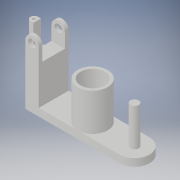
# Autodesk Inventor part: ValveBaseMk2.5
Saved by Autodesk Inventor 2019 (Build 230136000, 136)
## iProperties
Created: 2019-01-19
Part Number: ValveBaseMk2.5
Material: Generic
Document SubType Name: Modeling
Designer: Kepler
Density: 1 g/cm^3
Appearance: Default
Author: Kepler
Autodesk Inventor part; units mm, degrees
ref_plane "YZ Plane" through (0, 0, 0) normal (1, 0, 0) x (0, 1, 0)
ref_plane "XZ Plane" through (0, 0, 0) normal (0, 1, 0) x (-1, 0, 0)
ref_plane "XY Plane" through (0, 0, 0) normal (0, 0, 1) x (1, 0, 0)
sketch "Sketch1" plane through (0, 0, 0) normal (0, 0, 1) x (1, 0, 0)
  line L0 (0, 0) -> (0, 40)
  line L1 (0, 0) -> (63, 0)
  line L2 (63, 0) -> (63, 5)
  line L3 (63, 5) -> (9, 5)
  arc A0 (9, 40) -> (0, 40) centre (4.5, 40) ccw
  line L4 (9, 40) -> (9, 5)
  circle A1 centre (4.5, 40) radius 2.5
  dimension "d0" = 40
  dimension "d2" = 5
  dimension "d6" = 4.5
  dimension "d7" = 5
  dimension "d8" = 9
  dimension "d9" = 54
  dimension "d47" = 32.5
  constraints: 10 end point, 3 perpendicular, 2 centre point, 2 point on circle, 2 tangent, 1 coincident, 1 horizontal, 1 vertical
  measures "d0" distance of L0.start L0.end
  measures "d2" distance of L1.end L2.end
  measures "d6" radius of A0
  measures "d7" diameter of A1
  measures "d8" distance between parallel lines of L4 L0
  measures "d9" distance of L2.end L3.end
  measures "d47" distance edge to line of A1 L3
extrude "Extrusion1" add sketch "Sketch1" along normal blind 20
sketch "Sketch2" plane through (9, 5, 0) normal (0, 1, 0) x (1, 0, 0)
  line L0 (0, 0) -> (0, -20) projected
  circle A0 centre (26, -10) radius 10
  line L1 (0, 0) -> (54, 0) projected
  circle A1 centre (54, -10) radius 2.8
  line L2 (54, 0) -> (54, -20) projected
  point P0 (-9, 0)
  dimension "d14" = 20
  dimension "d16" = 26
  dimension "d20" = 5.6
  dimension "d21" = 10
  dimension "d22" = 15.2
  dimension "d67" = 0
  constraints: 2 centre point, 1 tangent
  measures "d14" diameter of A0
  measures "d16" distance from line of A0.centre L0
  measures "d20" diameter of A1
  measures "d21" distance from line of L1 A1.centre
  measures "d67" distance from line of L2 A1.centre
sketch "Sketch7" plane through (9, 5, 0) normal (1, 0, 0) x (0, 0, -1)
  line L0 (-10, 41.0364) -> (-10, 39.6436)
  line L1 (0, 39.5) -> (-20, 39.5) projected
  line L2 (-2.5, 39.5) -> (-2.5, 25.5)
  line L3 (-17.5, 39.5) -> (-17.5, 25.5)
  line L4 (-17.5, 39.5) -> (-2.5, 39.5)
  line L5 (0, 32.5) -> (-20, 32.5) projected
  line L6 (-17.5, 25.5) -> (-2.5, 25.5)
  point P0 (0, -5)
  dimension "d40" = 14
  dimension "d41" = 14
  dimension "d42" = 15
  constraints: 10 end point, 2 point on line, 2 vertical, 1 collinear, 1 perpendicular, 1 other
  measures "d40" distance of L2.start L2.end
  measures "d41" distance of L3.start L3.end
  measures "d42" distance between parallel lines of L3 L2
extrude "Extrusion5" cut sketch "Sketch7" against normal blind 14
extrude "Extrusion6" add sketch "Sketch2" along normal blind 25
sketch "Sketch9" plane through (35, 30, 10) normal (0, 1, 0) x (1, 0, 0)
  circle A0 centre (0, 0) radius 8
  point P0 (-35, 10)
  dimension "d50" = 16
  constraints: 1 centre point
  measures "d50" diameter of A0
extrude "Extrusion7" cut sketch "Sketch9" against normal blind 31
sketch "Sketch12" plane through (35, 5, 0) normal (0, 1, 0) x (1, 0, 0)
  line L0 (28, 0) -> (28, -20) projected
  arc A0 (28, -20) -> (28, 0) centre (28, -10) ccw
  line L1 (28, 0) -> (-35, 0) projected
  line L2 (28, 0) -> (28, -20)
  constraints: 2 end point, 2 point on circle, 1 centre point, 1 midpoint, 1 perpendicular
extrude "Extrusion10" add sketch "Sketch12" against normal blind 5
sketch "Sketch13" plane through (0, 0, 0) normal (0, -1, 0) x (1, 0, 0)
  circle A0 centre (-4, 10) radius 1
  line L0 (-4, 12.5) -> (0, 12.5)
  line L1 (0, 0) -> (0, 20) projected
  line L2 (-4, 7.5) -> (0, 7.5)
  arc A1 (-4, 12.5) -> (-4, 7.5) centre (-4, 10) ccw
  line L3 (0, 7.5) -> (0, 12.5)
  line L4 (63, 0) -> (0, 0) projected
  line L5 (0, 20) -> (63, 20) projected
  dimension "d68" = 2
  dimension "d72" = 4
  dimension "d73" = 10
  dimension "d74" = 20
  constraints: 6 end point, 2 centre point, 2 point on circle, 2 point on line, 2 tangent, 1 coincident, 1 collinear, 1 horizontal, 1 parallel
  measures "d68" diameter of A0
  measures "d72" distance from line of L1 A0.centre
  measures "d73" distance from line of L4 A0.centre
  measures "d74" distance between parallel lines of L5 L4
extrude "Extrusion11" add sketch "Sketch13" against normal blind 45
sketch "Sketch14" plane through (-4, 0, 12.5) normal (0, 0, 1) x (1, 0, 0)
  line L0 (0, 45) -> (4, 45) projected
  line L1 (13, 30.5) -> (4, 30.5) projected
  line L2 (4, 45) -> (4, 30.5)
  line L3 (4, 30.5) -> (2, 30.5)
  line L4 (2, 30.5) -> (2, 45)
  line L5 (2, 45) -> (4, 45)
  point P0 (4, 0)
  dimension "d75" = 2
  constraints: 8 end point, 4 perpendicular
  measures "d75" distance of L1.end L3.end
extrude "Extrusion12" cut sketch "Sketch14" against normal up to surface (5 mm away)
fillet "Fillet4" radius 2 1 edges at (-2, 30.5, 10)
equation "\"d21\" = d19"
equation "\"d40\" = d41"
equation "\"d73\" = 0.5 * d74"
equation "\"d19\" = 0.5 * d14"
body "Solid1"
